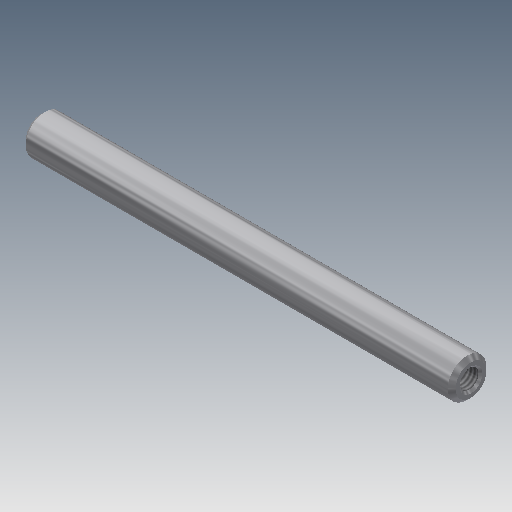
# Autodesk Inventor part: SETF5-55.5-M3-N3
Saved by Autodesk Inventor 2017.3 (Build 213256000, 256)
## iProperties
Category: PARTsolutions
Company: MISUMI
Created: 2016-05-27
Part Number: SETF5-55.5-M3-N3
Catalog Web Link: www.cadenas.de
Description: NETF, ETKF, PETF, SETF, AETTF-Circular Posts - Both Ends Tapped - Thread Diameter Configurable
Vendor: MISUMI
Document SubType Name: Modeling
Designer: psAdmin
Manufacturer: MISUMI
Mass: 8.03584 g
Surface Area: 10.2851 cm^2
Volume: 1.00448 cm^3
Density: 8 g/cm^3
Material: ステンレス鋼 AISI 304
Appearance: クローム - サテン
PSOL_IDENT_0: {$CADENAS_DATA\23d-libs\misumi\metric\19_posts_stands\petf.prj},232 {VTYP=3D},{NB=SETF5-55.5-M3-N3},
PSOL_IDENT_1: {LINA=SETF5-55.5-M3-N3},{NN=NETF, ETKF, PETF, SETF, AETTF},{DATE=18.11.2015 05:09:36},{GEOMDATE=30.1
PSOL_IDENT_2: 0.2015 07:35:48},{VERSION=},{LINEID=40},{LINESUBID=-1},{WBVAR=MAT,ST,M,N,ALT1,L,ALT2,HL,ALT4,ALT5}
PSOL_IDENT_3: {NB=SETF5-55.5-M3-N3},{LINA=SETF5-55.5-M3-N3},{KT=DUMMY},{PN=SETF5-55.5-M3-N3},{TYPE=SETF},{MAT=SUS3
PSOL_IDENT_4: 04},{MATALG= 'LCS', 'Low Carbon Steel', 'SUS304', 'SUS304' },{ST=-},{STALG= '-', '-' },{D=5},{M=3.0}
PSOL_IDENT_5: ,{M1=[2.6,3]},{MPITCH=0.500},{MDEPT=9.0},{MAV=3},{N=3.0},{N1=[2.6,3]},{NPITCH=0.500},{NDEPT=9.0},{NA
PSOL_IDENT_6: V=4},{ALT1=},{L=55.5},{LALG=[15:100/0.5]},{LMIN=15.0},{LMIN1=15},{LMIN2=13},{LMIN21=130},{LMIN22=150
PSOL_IDENT_7: },{LMIN23=150},{LMIN3=15},{LMAX=100},{ALT2=},{ALT2ALG='','Not applicable' },{ALT2PN=},{HL=0},{HLALG=
PSOL_IDENT_8: 0},{HLMIN=5},{HLMAX=50},{DD=0.0},{DD1=0.0},{ALT4=},{ALT4ALG='','w/o MD (Left End Change The Effectiv
PSOL_IDENT_9: e Tap Depth)','MD','with MD (Left End Change The Effective Tap Depth)'},{ALT4PN=-M3},{ALT5=},{ALT5AL
PSOL_IDENT_10: G='','w/o ND (Right End Change The Effective Tap Depth)','ND','with ND (Right End Change The Effecti
PSOL_IDENT_11: ve Tap Depth)'},{ALT5PN=-N3}
NN: NETF, ETKF, PETF, SETF, AETTF
NT: Circular Posts - Both Ends Tapped - Thread Diameter Configurable
NB: SETF5-55.5-M3-N3
NBSYN: $PN.
LINA: SETF5-55.5-M3-N3
PN: SETF5-55.5-M3-N3
MAT: SUS304
ST: -
D: 5
M: 3.0
N: 3.0
ALT1: w/o LKC (L Dimension Tolerance)
L: 55.5
ALT2: Not applicable
HL: 0
DD: 0.0
ALT4: w/o MD (Left End Change The Effective Tap Depth)
ALT5: w/o ND (Right End Change The Effective Tap Depth)
SUPPLIER: MISUMI
ARTICLENO: SETF5-55.5-M3-N3
BOMINFO: SETF5-55.5-M3-N3
CREATOR: CADENAS GmbH
Title: SETF5-55.5-M3-N3
Author: Cadenas PARTsolutions
Comments: Circular Posts - Both Ends Tapped - Thread Diameter Configurable
Autodesk Inventor part; units mm, degrees
ref_plane "YZ Plane" through (0, 0, 0) normal (1, 0, 0) x (0, 1, 0)
ref_plane "XZ Plane" through (0, 0, 0) normal (0, 1, 0) x (-1, 0, 0)
ref_plane "XY Plane" through (0, 0, 0) normal (0, 0, 1) x (1, 0, 0)
sketch "Sketch_1" plane through (0, 0, 0) normal (0, 0, 1) x (1, 0, 0)
  line L0 (55.5, 0) -> (0, 0)
  line L1 (0, 0) -> (0, 2)
  line L2 (0, 2) -> (0.5, 2.5)
  line L3 (0.5, 2.5) -> (55, 2.5)
  line L4 (55, 2.5) -> (55.5, 2)
  line L5 (55.5, 2) -> (55.5, 0)
  line L6 (55.5, 0) -> (0, 0)
  constraints: 14 end point
revolve "Revolution1" add sketch "Sketch_1" angle 360 about axis through (55.5, 0, 0) along (1, 0, 0)
sketch "Sketch2" plane through (0, 0, 0) normal (-1, 0, 0) x (0, 0, 1)
  point P0 (0, 0)
hole "Hole1" at (0, 0, 0) direction (1, 0, 0) diameter 2.459 depth 8.2901 tip angle 120 countersink diameter 3 countersink angle 90 thread size "M3x0.5" class "6H" standard "ISO Metric profile"
sketch "Sketch3" plane through (55.5, 0, 0) normal (1, 0, 0) x (0, 0, -1)
  point P0 (0, 0)
hole "Hole2" at (55.5, 0, 0) direction (-1, 0, 0) diameter 2.459 depth 8.2901 tip angle 120 countersink diameter 3 countersink angle 90 thread size "M3x0.5" class "6H" standard "ISO Metric profile"
body "Solid1"
